Autodesk Inventor part; units mm, degrees
(part 2 of 2)
sketch "Sketch22" plane through (-0.3992, -3.048, -545.9494) normal (-1, 0, 0) x (0, 0, 1)
  line L0 (367.1334, 0) -> (367.1334, -94.8254) projected
  line L1 (367.1334, -47.4127) -> (360.7834, -47.4127)
  line L2 (0, -94.8254) -> (367.1334, -94.8254) projected
  line L3 (360.7834, -94.8254) -> (360.7834, 0)
  line L4 (367.1334, 0) -> (0, 0) projected
  line L5 (0, 0) -> (0, -94.8254) projected
  line L6 (0, -47.4127) -> (6.35, -47.4127)
  line L7 (6.35, -94.8254) -> (6.35, 0)
  line L8 (183.5667, -94.8254) -> (183.5667, -88.4754)
  line L9 (183.5667, -88.4754) -> (360.7834, -88.4754)
  line L10 (183.5667, -88.4754) -> (6.35, -88.4754)
  line L11 (367.1334, 0) -> (367.1334, -6.35)
  line L12 (360.7834, -6.35) -> (6.35, -6.35)
  line L13 (6.35, -88.4754) -> (65.405, -88.4754)
  circle A0 centre (65.405, -88.4754) radius 6.35
  line L14 (65.405, -88.4754) -> (183.5667, -88.4754)
  line L15 (65.405, -88.4754) -> (183.5667, -88.4754)
  line L16 (124.4859, -88.4754) -> (124.4859, -47.4036)
  circle A1 centre (124.4859, -47.4036) radius 6.35
  line L17 (65.405, -88.4754) -> (124.4859, -47.4036) construction
  line L18 (65.405, -88.4754) -> (6.35, -47.4127) construction
  line L19 (124.4859, -47.4036) -> (6.35, -47.4127) construction
  line L20 (62.6862, -92.3855) -> (68.1238, -84.5652)
  line L21 (68.1238, -84.5652) -> (9.0688, -43.5025)
  line L22 (9.0688, -43.5025) -> (3.6312, -51.3228)
  line L23 (3.6312, -51.3228) -> (68.1238, -84.5652) construction
  line L24 (62.6862, -92.3855) -> (9.0688, -43.5025) construction
  line L25 (121.7674, -43.4932) -> (62.6866, -84.565)
  line L26 (62.6866, -84.565) -> (68.1234, -92.3858)
  line L27 (68.1234, -92.3858) -> (127.2043, -51.314)
  line L28 (127.2043, -51.314) -> (121.7674, -43.4932)
  line L29 (121.7674, -43.4932) -> (68.1234, -92.3858) construction
  line L30 (62.6866, -84.565) -> (127.2043, -51.314) construction
  line L31 (65.405, -94.8254) -> (65.4051, -83.1639)
  line L32 (124.4855, -42.6411) -> (6.3496, -42.6502)
  line L33 (6.3496, -42.6502) -> (6.3504, -52.1752)
  line L34 (6.3504, -52.1752) -> (124.4862, -52.1661)
  line L35 (124.4862, -52.1661) -> (124.4855, -42.6411)
  line L36 (124.4855, -42.6411) -> (6.3504, -52.1752) construction
  line L37 (6.3496, -42.6502) -> (124.4862, -52.1661) construction
  line L38 (109.2899, -52.1673) -> (65.4053, -82.675)
  line L39 (21.5399, -52.174) -> (65.4053, -82.675)
  line L40 (21.5399, -52.174) -> (109.2899, -52.1673)
  circle A2 centre (183.5667, -88.4754) radius 6.35
  circle A3 centre (183.5667, -6.35) radius 6.35
  line L41 (360.7834, -88.4754) -> (301.7284, -88.4754)
  line L42 (301.7284, -88.4754) -> (183.5667, -88.4754)
  circle A4 centre (242.6476, -47.4036) radius 6.35
  circle A5 centre (301.7284, -88.4754) radius 6.35
  circle A6 centre (301.6984, -6.347) radius 6.35
  line L43 (242.6476, -47.4036) -> (183.5667, -88.4754) construction
  line L44 (124.4859, -47.4036) -> (183.5667, -88.4754) construction
  line L45 (124.4859, -47.4036) -> (242.6476, -47.4036) construction
  line L46 (242.6476, -42.6411) -> (124.4859, -42.6411) construction
  line L47 (124.4859, -42.6411) -> (124.4859, -52.1661) construction
  line L48 (124.4859, -52.1661) -> (242.6476, -52.1661) construction
  line L49 (242.6476, -52.1661) -> (242.6476, -42.6411) construction
  line L50 (242.6476, -42.6411) -> (124.4859, -52.1661) construction
  line L51 (124.4859, -42.6411) -> (242.6476, -52.1661) construction
  line L52 (239.9291, -43.4932) -> (180.8483, -84.565) construction
  line L53 (180.8483, -84.565) -> (186.2852, -92.3858) construction
  line L54 (186.2852, -92.3858) -> (245.366, -51.314) construction
  line L55 (245.366, -51.314) -> (239.9291, -43.4932) construction
  line L56 (239.9291, -43.4932) -> (186.2852, -92.3858) construction
  line L57 (180.8483, -84.565) -> (245.366, -51.314) construction
  line L58 (121.7674, -51.314) -> (180.8483, -92.3858) construction
  line L59 (180.8483, -92.3858) -> (186.2852, -84.565) construction
  line L60 (186.2852, -84.565) -> (127.2043, -43.4932) construction
  line L61 (127.2043, -43.4932) -> (121.7674, -51.314) construction
  line L62 (121.7674, -51.314) -> (186.2852, -84.565) construction
  line L63 (180.8483, -92.3858) -> (127.2043, -43.4932) construction
  line L64 (227.4533, -52.1661) -> (183.5667, -82.6752)
  line L65 (183.5667, -82.6752) -> (139.6801, -52.1661)
  line L66 (139.6801, -52.1661) -> (227.4533, -52.1661)
  line L67 (175.2232, -88.4754) -> (124.4859, -53.2038)
  line L68 (175.2232, -88.4754) -> (73.7485, -88.4754)
  line L69 (301.7284, -88.4754) -> (242.6476, -47.4036) construction
  line L70 (301.6984, -6.347) -> (242.6491, -47.4057) construction
  line L71 (301.6984, -6.347) -> (360.7834, -47.4127) construction
  line L72 (360.7834, -47.4127) -> (301.7284, -88.4754) construction
  line L73 (239.9291, -51.314) -> (299.01, -92.3858) construction
  line L74 (299.01, -92.3858) -> (304.4469, -84.565) construction
  line L75 (304.4469, -84.565) -> (245.366, -43.4932) construction
  line L76 (245.366, -43.4932) -> (239.9291, -51.314) construction
  line L77 (239.9291, -51.314) -> (304.4469, -84.565) construction
  line L78 (299.01, -92.3858) -> (245.366, -43.4932) construction
  line L79 (358.0646, -43.5025) -> (299.0096, -84.5652) construction
  line L80 (299.0096, -84.5652) -> (304.4473, -92.3855) construction
  line L81 (304.4473, -92.3855) -> (363.5023, -51.3228) construction
  line L82 (363.5023, -51.3228) -> (358.0646, -43.5025) construction
  line L83 (358.0646, -43.5025) -> (304.4473, -92.3855) construction
  line L84 (299.0096, -84.5652) -> (363.5023, -51.3228) construction
  line L85 (363.4992, -43.5004) -> (304.4187, -2.4379) construction
  line L86 (304.4187, -2.4379) -> (298.9826, -10.2593) construction
  line L87 (298.9826, -10.2593) -> (358.0631, -51.3218) construction
  line L88 (358.0631, -51.3218) -> (363.4992, -43.5004) construction
  line L89 (363.4992, -43.5004) -> (298.9826, -10.2593) construction
  line L90 (304.4187, -2.4379) -> (358.0631, -51.3218) construction
  line L91 (242.6433, -47.4098) -> (360.7877, -47.4189) construction
  line L92 (242.6476, -42.6518) -> (360.7834, -42.6518) construction
  line L93 (360.7834, -42.6518) -> (360.7834, -52.1768) construction
  line L94 (360.7834, -52.1768) -> (242.6476, -52.1768) construction
  line L95 (242.6476, -52.1768) -> (242.6476, -42.6518) construction
  line L96 (242.6476, -42.6518) -> (360.7834, -52.1768) construction
  line L97 (360.7834, -42.6518) -> (242.6476, -52.1768) construction
  line L98 (298.989, -2.4303) -> (239.9208, -43.5022) construction
  line L99 (239.9208, -43.5022) -> (245.3585, -51.3225) construction
  line L100 (245.3585, -51.3225) -> (304.4267, -10.2506) construction
  line L101 (304.4267, -10.2506) -> (298.989, -2.4303) construction
  line L102 (298.989, -2.4303) -> (245.3585, -51.3225) construction
  line L103 (239.9208, -43.5022) -> (304.4267, -10.2506) construction
  line L104 (183.5667, -6.35) -> (242.6433, -47.4098) construction
  line L105 (183.5667, -6.35) -> (124.4859, -47.4036) construction
  circle A7 centre (65.418, -6.3498) radius 6.35
  line L106 (124.4859, -47.4036) -> (65.418, -6.3498) construction
  line L107 (65.418, -6.3498) -> (6.35, -47.4127) construction
  line L108 (186.2848, -2.4393) -> (245.3613, -43.4991) construction
  line L109 (245.3613, -43.4991) -> (239.9252, -51.3205) construction
  line L110 (239.9252, -51.3205) -> (180.8487, -10.2607) construction
  line L111 (180.8487, -10.2607) -> (186.2848, -2.4393) construction
  line L112 (186.2848, -2.4393) -> (239.9252, -51.3205) construction
  line L113 (245.3613, -43.4991) -> (180.8487, -10.2607) construction
  line L114 (180.844, -2.4334) -> (121.7717, -43.4993) construction
  line L115 (121.7717, -43.4993) -> (127.2086, -51.3202) construction
  line L116 (127.2086, -51.3202) -> (186.2809, -10.2543) construction
  line L117 (186.2809, -10.2543) -> (180.844, -2.4334) construction
  line L118 (180.844, -2.4334) -> (127.2086, -51.3202) construction
  line L119 (121.7717, -43.4993) -> (186.2809, -10.2543) construction
  line L120 (360.7834, -88.4754) -> (310.0707, -88.4754)
  line L121 (360.7834, -53.2133) -> (360.7834, -88.4754)
  line L122 (360.7834, -41.6129) -> (360.7834, -6.35)
  line L123 (360.7834, -6.35) -> (310.0474, -6.35)
  line L124 (360.7834, -88.4754) -> (360.7834, -53.2133)
  line L125 (242.6476, -53.2038) -> (191.9102, -88.4754)
  line L126 (293.3849, -88.4754) -> (242.6476, -53.2038)
  line L127 (293.3849, -88.4754) -> (191.9102, -88.4754)
  line L128 (345.5888, -42.6518) -> (301.699, -12.1472)
  line L129 (301.699, -12.1472) -> (257.8283, -42.6518)
  line L130 (257.8283, -42.6518) -> (345.5888, -42.6518)
  line L131 (191.9115, -6.35) -> (293.401, -6.35)
  line L132 (227.4374, -42.6411) -> (183.5605, -12.1455)
  line L133 (183.5605, -12.1455) -> (139.6932, -42.6411)
  line L134 (139.6932, -42.6411) -> (227.4374, -42.6411)
  line L135 (127.2121, -43.4986) -> (68.1278, -2.4335) construction
  line L136 (68.1278, -2.4335) -> (62.6918, -10.2549) construction
  line L137 (62.6918, -10.2549) -> (121.776, -51.32) construction
  line L138 (121.776, -51.32) -> (127.2121, -43.4986) construction
  line L139 (127.2121, -43.4986) -> (62.6918, -10.2549) construction
  line L140 (68.1278, -2.4335) -> (121.776, -51.32) construction
  line L141 (62.6995, -2.4394) -> (3.6316, -43.5023) construction
  line L142 (3.6316, -43.5023) -> (9.0685, -51.3231) construction
  line L143 (9.0685, -51.3231) -> (68.1364, -10.2603) construction
  line L144 (68.1364, -10.2603) -> (62.6995, -2.4394) construction
  line L145 (62.6995, -2.4394) -> (9.0685, -51.3231) construction
  line L146 (3.6316, -43.5023) -> (68.1364, -10.2603) construction
  line L147 (175.2101, -6.35) -> (73.7629, -6.35)
  line L148 (6.35, -41.6125) -> (6.35, -6.35)
  line L149 (6.35, -6.35) -> (57.0743, -6.35)
  line L150 (109.2905, -42.6423) -> (65.4163, -12.1513)
  line L151 (65.4163, -12.1513) -> (21.5459, -42.649)
  line L152 (109.2905, -42.6423) -> (21.5459, -42.649)
  line L153 (57.0627, -88.4754) -> (6.35, -88.4754)
  line L154 (6.35, -52.7243) -> (6.35, -88.4754)
  line L155 (6.35, -53.2133) -> (6.35, -88.4754)
  line L156 (345.5895, -52.1768) -> (301.7281, -82.675)
  line L157 (301.7281, -82.675) -> (257.8573, -52.1768)
  line L158 (257.8573, -52.1768) -> (345.5895, -52.1768)
  line L159 (310.0707, -88.4754) -> (360.7834, -88.4754)
  line L160 (367.1334, -88.4754) -> (0, -88.4754)
  line L161 (367.1334, -6.35) -> (0, -6.35)
  line L162 (370.3084, -9.525) -> (370.3084, 0)
  line L163 (52.5071, -9.525) -> (9.525, -39.4053)
  line L164 (9.525, -9.525) -> (9.525, -39.4053)
  line L165 (9.525, -9.525) -> (52.5071, -9.525)
  line L166 (357.6084, -39.4062) -> (357.6084, -9.525)
  line L167 (314.6156, -9.525) -> (357.6084, -9.525)
  line L168 (314.6156, -9.525) -> (357.6084, -39.4062)
  line L169 (357.6084, -85.3004) -> (314.6369, -85.3004)
  line L170 (357.6084, -55.421) -> (314.6369, -85.3004)
  line L171 (357.6084, -55.421) -> (357.6084, -85.3004)
  line L172 (288.8178, -85.3004) -> (196.4774, -85.3004)
  line L173 (288.8178, -85.3004) -> (242.6476, -53.2038)
  line L174 (242.6476, -53.2038) -> (196.4774, -85.3004)
  line L175 (170.656, -85.3004) -> (78.3157, -85.3004)
  line L176 (78.3157, -85.3004) -> (124.4859, -53.2038)
  line L177 (124.4859, -53.2038) -> (170.656, -85.3004)
  line L178 (52.4965, -85.3004) -> (9.525, -55.421)
  line L179 (9.525, -85.3004) -> (9.525, -55.421)
  line L180 (9.525, -85.3004) -> (52.4965, -85.3004)
  line L181 (9.525, -39.4053) -> (9.525, -9.525)
  line L182 (9.525, -9.525) -> (52.5071, -9.525)
  line L183 (52.5071, -9.525) -> (9.525, -39.4053)
  line L184 (196.4796, -9.525) -> (242.6427, -41.6095)
  line L185 (242.6427, -41.6095) -> (288.83, -9.525)
  line L186 (288.83, -9.525) -> (196.4796, -9.525)
  line L187 (314.6156, -9.525) -> (357.6084, -39.4062)
  line L188 (357.6084, -39.4062) -> (357.6084, -9.525)
  line L189 (357.6084, -9.525) -> (314.6156, -9.525)
  line L190 (357.6084, -39.4062) -> (314.6156, -9.525)
  line L191 (314.6156, -9.525) -> (357.6084, -9.525)
  line L192 (288.8178, -85.3004) -> (196.4774, -85.3004)
  line L193 (242.6476, -53.2038) -> (196.4774, -85.3004)
  line L194 (242.6476, -53.2038) -> (288.8178, -85.3004)
  line L195 (357.6084, -55.421) -> (314.6369, -85.3004)
  line L196 (314.6369, -85.3004) -> (357.6084, -85.3004)
  line L197 (357.6084, -55.421) -> (357.6084, -85.3004)
  line L198 (345.5895, -52.1768) -> (301.7281, -82.675)
  line L199 (301.7281, -82.675) -> (257.8573, -52.1768)
  line L200 (257.8573, -52.1768) -> (345.5895, -52.1768)
  line L201 (124.4859, -9.525) -> (170.6429, -9.525)
  line L202 (124.4859, -9.525) -> (78.3311, -9.525)
  line L203 (78.3311, -9.525) -> (124.4921, -41.6081)
  line L204 (124.4921, -41.6081) -> (170.6429, -9.525)
  line L205 (367.1334, -94.8254) -> (360.7834, -94.8254)
  line L206 (360.7834, -94.8254) -> (360.7834, -88.4754)
  line L207 (360.7834, -88.4754) -> (367.1334, -88.4754)
  line L208 (367.1334, -88.4754) -> (367.1334, -94.8254)
  line L209 (367.1334, 0) -> (360.7834, 0)
  line L210 (360.7834, 0) -> (360.7834, -6.35)
  line L211 (360.7834, -6.35) -> (367.1334, -6.35)
  line L212 (367.1334, -6.35) -> (367.1334, 0)
  line L213 (0, 0) -> (6.35, 0)
  line L214 (6.35, 0) -> (6.35, -6.35)
  line L215 (6.35, -6.35) -> (0, -6.35)
  line L216 (0, -6.35) -> (0, 0)
  line L217 (0, -94.8254) -> (6.35, -94.8254)
  line L218 (6.35, -94.8254) -> (6.35, -88.4754)
  line L219 (6.35, -88.4754) -> (0, -88.4754)
  line L220 (0, -88.4754) -> (0, -94.8254)
  arc A8 (11.8493, -85.3004) -> (9.525, -82.9761) centre (6.35, -88.4754) ccw
  arc A9 (357.6084, -82.9761) -> (355.2842, -85.3004) centre (360.7834, -88.4754) ccw
  arc A10 (9.525, -11.8493) -> (11.8493, -9.525) centre (6.35, -6.35) ccw
  arc A11 (6.35, 0) -> (6.3463, 0) centre (6.35, -6.35) ccw
  arc A12 (355.2842, -9.525) -> (357.6084, -11.8493) centre (360.7834, -6.35) ccw
  point P0 (545.9494, 3.048)
  point P1 (35.8775, -67.944)
  point P2 (94.9454, -67.9395)
  point P3 (65.4179, -47.4081)
  point P4 (183.5667, -47.4036)
  point P5 (213.1072, -67.9395)
  point P6 (154.0263, -67.9395)
  point P7 (272.188, -67.9395)
  point P8 (331.2559, -67.944)
  point P9 (331.2409, -26.8799)
  point P10 (301.7155, -47.4143)
  point P11 (272.1737, -26.8764)
  point P12 (213.105, -26.8799)
  point P13 (154.0263, -26.8768)
  point P14 (94.9519, -26.8767)
  point P15 (35.884, -26.8813)
  point P16 (357.6084, -82.9761)
  point P17 (355.2842, -9.525)
  point P18 (357.6084, -11.8493)
  point P19 (9.525, -11.8493)
  point P20 (11.8493, -9.525)
  dimension "d443" = 12.7
  dimension "MinimumRemnant" = 6.096
  dimension "d438" = 6.35
  dimension "d439" = 6.35
  dimension "d440" = 6.35
  dimension "d441" = 6.35
  dimension "d442" = 59.055
  dimension "d444" = 41.0718
  dimension "d445" = 12.7
  dimension "d446" = 9.525
  dimension "d447" = 9.525
  dimension "d448" = 9.525
  dimension "d451" = 59.055
  dimension "d453" = 12.7
  dimension "d454" = 12.7
  dimension "d455" = 12.7
  dimension "d456" = 9.525
  dimension "d457" = 9.525
  dimension "d458" = 9.525
  dimension "d461" = 9.525
  dimension "d462" = 9.525
  dimension "d463" = 9.525
  dimension "d464" = 9.525
  dimension "d465" = 9.525
  dimension "d466" = 12.7
  dimension "d467" = 9.525
  dimension "d468" = 9.525
  dimension "d469" = 9.525
  dimension "d470" = 9.525
  constraints: 432 end point, 105 point on line, 51 parallel, 49 midpoint, 29 perpendicular, 28 collinear, 11 centre point, 10 point on circle, 9 horizontal, 8 coincident, 4 vertical, 2 vertical alignment, 14 other
  measures "d438" distance of L1.start L1.end
  measures "d439" distance of L6.start L6.end
  measures "d440" distance of L8.start L8.end
  measures "d441" distance of L11.end L0.start
  measures "d442" distance of L10.end L13.end
  measures "d444" distance of L16.start L16.end
  measures "d445" diameter of A1
  measures "d446" distance of L20.end L20.start
  measures "d447" distance of L26.end L25.end
  measures "d448" distance of L33.end L32.end
  measures "d451" distance of L9.end L41.end
  measures "d453" diameter of A4
  measures "d454" diameter of A5
  measures "d455" diameter of A6
  measures "d456" distance of L47.end L46.end
  measures "d457" distance of L53.end L52.end
  measures "d458" distance of L59.end L58.end
  measures "d461" distance of L74.end L73.end
  measures "d462" distance of L80.end L79.end
  measures "d463" distance of L86.end L85.end
  measures "d464" distance of L92.end L93.end
  measures "d465" distance of L99.end L98.end
  measures "d466" diameter of A7
  measures "d467" distance of L108.end L109.end
  measures "d468" distance of L115.end L114.end
  measures "d469" distance of L136.end L135.end
  measures "d470" distance of L142.end L141.end
extrude "Cut5" cut sketch "Sketch22" against normal blind 3.048 contours L128 L130 L129 A6 | A6 L129 L128 | L132 L134 L133 A3 | A3 L133 L132 | L156 L157 A5 | A5 L157 L158 L156 | L150 L32 L151 A7 | A7 L151 L150 | L64 L65 A2 | A2 L65 L66 L64 | L172 L125 A4 L126 | L21 L34 L25 A0 | A0 L25 L21 | L175 L16 A1 L67 | A4 L125 L126 | L203 L202 L201 L204 A1 | A1 L204 L203 | L27 A1 L16 L175 | A1 L16 L67 | L27 L16 A1 | L184 L186 L185 A4 | A4 L185 L184 | L163 L164 A10 L165 | A10 L164 L165 | L168 L167 A12 L166 | A12 L167 L166 | L169 A9 L171 | L169 L170 L171 A9 | L180 A8 L179 L178
hole "Hole6" at (-0.3992, -91.5234, -185.166) at (-0.3992, -91.5234, -244.221) at (-0.3992, -9.395, -244.2511) at (-0.3992, -9.398, -185.166) at (-0.3992, -50.4537, -303.3004) at (-0.3992, -91.5234, -362.3827) at (-0.3992, -9.398, -362.3827) at (-0.3992, -50.4516, -421.4636) at (-0.3992, -91.5234, -480.5444) at (-0.3992, -9.3978, -480.5315) at (-0.3992, -91.5234, -539.5994) at (-0.3992, -9.398, -539.5994) direction (1, 0, 0) diameter 6.604 end through all
extrude "Extrusion2" add sketch "Sketch22" against normal up to surface (3.048 mm away) contours A10 L164 L165 | A12 L167 L166 | L169 A9 L171
sketch "Sketch11" plane through (5.6968, -100.9214, -178.816) normal (0, -1, 0) x (-1, 0, 0)
  line L0 (0, -367.1334) -> (0, 0)
  line L1 (0, 0) -> (-19.304, 0)
  line L2 (-19.304, 0) -> (-19.304, -367.1334)
  line L3 (-19.304, -367.1334) -> (0, -367.1334)
  constraints: 6 end point, 1 horizontal, 1 perpendicular, 1 vertical
sketch "Sketch12" plane through (5.6968, -97.8734, -548.9974) normal (0, 0, -1) x (1, 0, 0)
  line L0 (0, 6.3246) -> (0, 0)
  line L1 (0, 0) -> (19.304, 0)
  line L2 (19.304, 0) -> (19.304, 6.3246)
  line L3 (19.304, 6.3246) -> (0, 6.3246)
  constraints: 6 end point, 1 horizontal, 1 perpendicular, 1 vertical
sketch "Sketch14" plane through (5.6968, -3.048, -175.768) normal (0, 0, 1) x (-1, 0, 0)
  line L0 (0, -94.8254) -> (0, 0)
  line L1 (0, 0) -> (-19.304, 0)
  line L2 (-19.304, 0) -> (-19.304, -94.8254)
  line L3 (-19.304, -94.8254) -> (0, -94.8254)
  constraints: 6 end point, 1 horizontal, 1 perpendicular, 1 vertical
equation "\"d35\" = Thickness"
equation "\"d44\" = BendReliefWidth"
equation "\"d45\" = BendReliefDepth"
equation "\"d46\" = MinimumRemnant"
equation "\"d47\" = TransitionRadius"
equation "\"d49\" = BendRadius"
equation "\"d56\" = BendReliefWidth"
equation "\"d57\" = BendReliefDepth"
equation "\"d58\" = MinimumRemnant"
equation "\"d59\" = TransitionRadius"
equation "\"d61\" = BendRadius"
equation "\"d62\" = BendReliefWidth"
equation "\"d63\" = BendReliefDepth"
equation "\"d64\" = MinimumRemnant"
equation "\"d65\" = TransitionRadius"
equation "\"d67\" = BendRadius"
equation "\"d79\" = BendReliefWidth"
equation "\"d80\" = BendReliefDepth"
equation "\"d81\" = MinimumRemnant"
equation "\"d82\" = TransitionRadius"
equation "\"d84\" = BendRadius"
equation "\"MinimumRemnant\" = 2 * Thickness"
equation "\"d39\" = BendRadius"
equation "\"d40\" = BendReliefWidth"
equation "\"d42\" = MinimumRemnant"
equation "\"d41\" = BendReliefDepth"
equation "\"d43\" = TransitionRadius"
equation "\"BendRadius\" = Thickness"
equation "\"BendReliefWidth\" = Thickness"
equation "\"BendReliefDepth\" = 0.5 * Thickness"
equation "\"CornerReliefSize\" = 4 * Thickness"
equation "\"TransitionRadius\" = BendRadius"
equation "\"JacobiRadiusSize\" = BendRadius"
equation "\"GapSize\" = Thickness"
equation "\"Thickness\" = 3.048"
body "Solid1"
